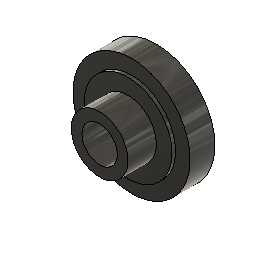
Center v1 (Autodesk Fusion 360 design; units mm, degrees)
Autodesk Fusion 360 part; units mm, degrees
sketch "Sketch1" plane through (0, 0, 0) normal (0, 0, 1) x (1, 0, 0)
  circle A0 centre (0, 0) radius 6.2
  circle A1 centre (0, 0) radius 4
  circle A2 centre (0, 0) radius 2.5
  circle A3 centre (0, 0) radius 8.25
  dimension "d1" = 12.4
  dimension "d2" = 8
  dimension "d3" = 5
  dimension "d4" = 16.5
  measures "d1" diameter of A0
  measures "d2" diameter of A1
  measures "d3" diameter of A2
  measures "d4" diameter of A3
extrude "Extrude1" add sketch "Sketch1" along normal blind 8 contours A1
extrude "Extrude2" add sketch "Sketch1" along normal blind 3.5 contours A0 | A3
extrude "Extrude3" add sketch "Sketch1" along normal blind 0.5 from surface at 3.5 contours A0
sketch "Sketch2" plane through (0, 0, 0) normal (0, 0, 1) x (1, 0, 0)
  circle A0 centre (0, 0) radius 8.25
  circle A1 centre (0, 0) radius 2.5
  circle A2 centre (0, 0) radius 6.2
  circle A3 centre (0, 0) radius 4
